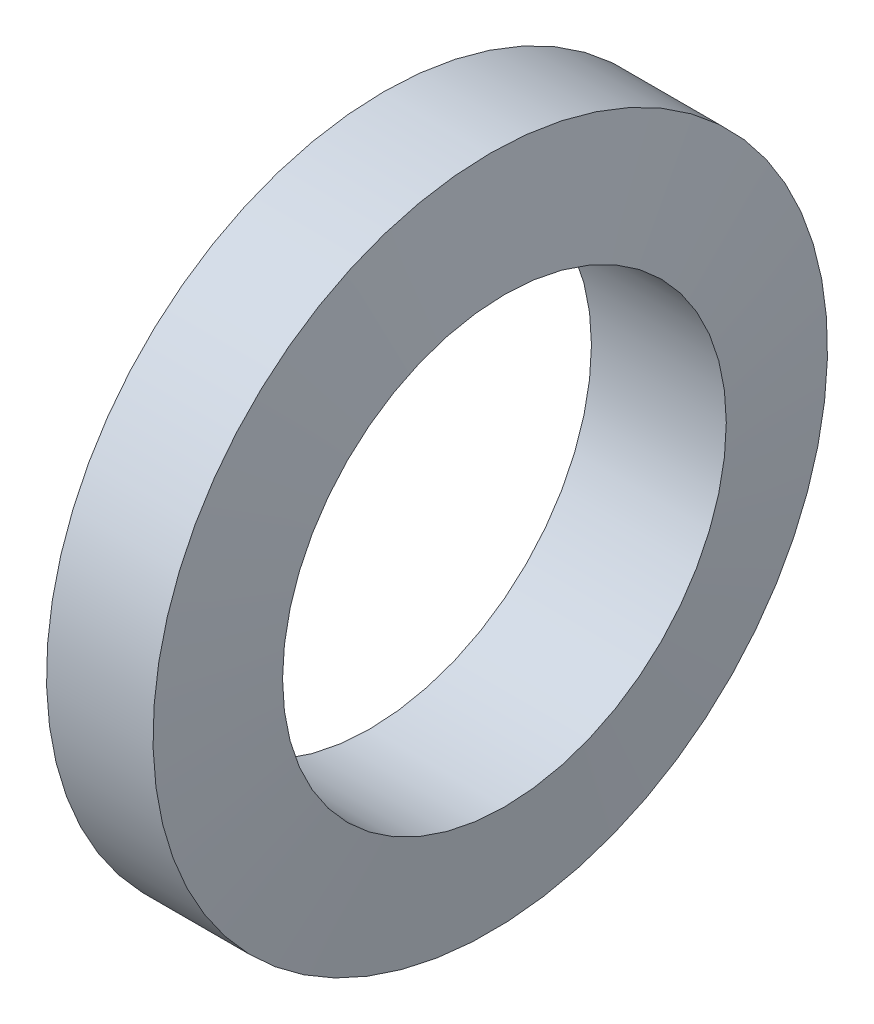
# Autodesk Inventor part: 高速轴油封
Saved by Autodesk Inventor 2025 (Build 290162000, 162)
## iProperties
Created: 2025-03-19
Part Number: 高速轴油封
Material: 常规
Document SubType Name: Modeling
Designer: liukan
Density: 1 g/cm^3
Appearance: 默认
Author: liukan
Autodesk Inventor part; units mm, degrees
ref_plane "YZ Plane" through (0, 0, 0) normal (1, 0, 0) x (0, 1, 0)
ref_plane "XZ Plane" through (0, 0, 0) normal (0, 1, 0) x (-1, 0, 0)
ref_plane "XY Plane" through (0, 0, 0) normal (0, 0, 1) x (1, 0, 0)
sketch "草图2" plane through (0, 0, 0) normal (0, 0, 1) x (1, 0, 0)
  line L0 (4.5, 19) -> (3.7633, 13)
  line L1 (4.5, 19) -> (10.5, 19) projected
  line L2 (11.2367, 13) -> (10.5, 19)
  line L3 (10.5, 19) -> (4.5, 19)
  line L4 (4.5, 19) -> (3.7019, 12.5)
  line L5 (3.7019, 12.5) -> (11.2981, 12.5)
  line L6 (11.2981, 12.5) -> (10.5, 19)
  line L7 (0, 0) -> (15.5876, 0) construction
  dimension "d3" = 12.5
  constraints: 14 end point, 3 horizontal, 1 collinear, 1 point on line, 5 other
  measures "d3" distance from line of L7.start L5
revolve "旋转2" add sketch "草图2" angle 360 about axis through (0, 0, 0) along (1, 0, 0)
